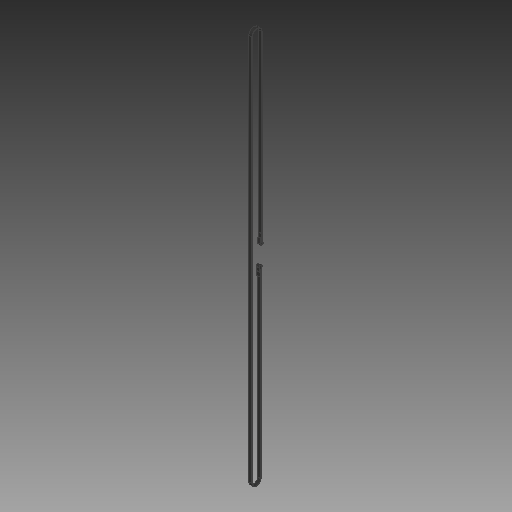
# Autodesk Inventor part: first stage belt
Saved by Autodesk Inventor 2017 SP1 (Build 210196100, 196)
## iProperties
Created: 2018-01-21
Part Number: first stage belt
Material: Rubber
Document SubType Name: Modeling
Designer: Ben
Density: 0.93 g/cm^3
Appearance: Rubber - Black
Mass: 35.134 g
Surface Area: 555.576 cm^2
Volume: 37.7784 cm^3
Author: Ben
Autodesk Inventor part; units mm, degrees
ref_plane "YZ Plane" through (0, 0, 0) normal (1, 0, 0) x (0, 1, 0)
ref_plane "XZ Plane" through (0, 0, 0) normal (0, 1, 0) x (-1, 0, 0)
ref_plane "XY Plane" through (0, 0, 0) normal (0, 0, 1) x (1, 0, 0)
sketch "Sketch1" plane through (0, 0, 0) normal (1, 0, 0) x (0, 1, 0)
  line L0 (596.9, 0) -> (-596.9, 0)
  line L1 (0, 0) -> (0, -26.9875) construction
  arc A0 (596.9, -28.575) -> (596.9, 0) centre (596.9, -14.2875) ccw
  line L2 (596.9, -28.575) -> (45.0045, -28.575)
  arc A1 (-596.9, 0) -> (-596.9, -25.4) centre (-596.9, -12.7) ccw
  line L3 (-596.9, -25.4) -> (-45.0045, -25.4)
  arc A2 (30.8471, -25.4747) -> (30.8765, -31.6687) centre (30.1625, -28.575) ccw
  arc A3 (-30.8765, -28.4937) -> (-30.8471, -22.2997) centre (-30.1625, -25.4) ccw
  line L4 (45.0045, -30.1625) -> (596.9, -30.1625)
  arc A4 (596.9, -30.1625) -> (596.9, 1.5875) centre (596.9, -14.2875) ccw
  line L5 (596.9, 1.5875) -> (-596.9, 1.5875)
  arc A5 (-596.9, 1.5875) -> (-596.9, -26.9875) centre (-596.9, -12.7) ccw
  line L6 (-596.9, -26.9875) -> (-45.0045, -26.9875)
  line L7 (30.1625, -28.575) -> (-30.1625, -25.4) construction
  arc A6 (31.1894, -23.9245) -> (31.2335, -33.2155) centre (30.1625, -28.575) ccw
  arc A7 (45.0045, -28.575) -> (43.5765, -28.7376) centre (45.0045, -34.925) ccw
  line L8 (43.5765, -28.7376) -> (30.8765, -31.6687)
  arc A8 (45.0045, -30.1625) -> (43.9335, -30.2845) centre (45.0045, -34.925) ccw
  line L9 (43.9335, -30.2845) -> (31.2335, -33.2155)
  arc A9 (43.6352, -28.2986) -> (45.0045, -28.448) centre (45.0045, -22.098) ccw
  line L10 (45.0045, -28.448) -> (57.7045, -28.448)
  line L11 (43.6352, -28.2986) -> (30.8471, -25.4747)
  line L12 (45.0045, -28.448) -> (45.0045, -28.575) construction
  line L13 (57.7045, -28.448) -> (57.7045, -26.8605)
  line L14 (57.7045, -26.8605) -> (45.0045, -26.8605)
  arc A10 (43.9775, -26.7485) -> (45.0045, -26.8605) centre (45.0045, -22.098) ccw
  line L15 (43.9775, -26.7485) -> (31.1894, -23.9245)
  arc A11 (-43.9335, -27.1095) -> (-45.0045, -26.9875) centre (-45.0045, -31.75) ccw
  arc A12 (-43.5765, -25.5626) -> (-45.0045, -25.4) centre (-45.0045, -31.75) ccw
  line L16 (-43.5765, -25.5626) -> (-30.8765, -28.4937)
  arc A13 (-31.2335, -30.0405) -> (-31.1894, -20.7495) centre (-30.1625, -25.4) ccw
  line L17 (-31.2335, -30.0405) -> (-43.9335, -27.1095)
  line L18 (-30.8471, -22.2997) -> (-43.6352, -25.1236)
  arc A14 (-45.0045, -25.273) -> (-43.6352, -25.1236) centre (-45.0045, -18.923) ccw
  line L19 (-45.0045, -25.4) -> (-45.0045, -25.273) construction
  line L20 (-45.0045, -25.273) -> (-57.7045, -25.273)
  line L21 (-57.7045, -25.273) -> (-57.7045, -23.6855)
  line L22 (-57.7045, -23.6855) -> (-45.0045, -23.6855)
  arc A15 (-45.0045, -23.6855) -> (-43.9775, -23.5735) centre (-45.0045, -18.923) ccw
  line L23 (-43.9775, -23.5735) -> (-31.1894, -20.7495)
  dimension "d1" = 14.2875
  dimension "d2" = 12.7
  dimension "d4" = 6.35
  dimension "d5" = 1.5875
  dimension "d6" = 60.325
  dimension "d7" = 6.35
  dimension "d8" = 12.7
  dimension "d9" = 12.7
  dimension "d10" = 0.127
  dimension "d11" = 6.35
  dimension "d12" = 12.7
  dimension "d13" = 0.127
  dimension "d14" = 12.7
  dimension "d15" = 1193.8
  constraints: 49 end point, 32 point on circle, 26 tangent, 16 centre point, 7 coincident, 6 parallel, 5 horizontal, 5 vertical, 3 equal radius, 2 midpoint, 2 point on line, 1 line through centre, 1 perpendicular, 4 other
  measures "d1" radius of A0
  measures "d2" radius of A1
  measures "d4" diameter of A2
  measures "d5" distance between parallel lines of L5 L0
  measures "d6" horizontal distance of L7.start L7.end
  measures "d7" radius of A7
  measures "d8" horizontal distance of L8.start L8.end
  measures "d9" distance of L10.start L10.end
  measures "d10" distance between parallel lines of L10 L2
  measures "d11" radius of A12
  measures "d12" horizontal distance of L16.start L16.end
  measures "d13" distance of L3.end L19.end
  measures "d14" distance of L19.end L20.end
  measures "d15" distance of A1.centre A0.centre
extrude "Extrusion1" add sketch "Sketch1" along normal mid plane 9.525
body "Solid1"
